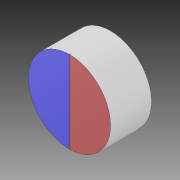
# Autodesk Inventor part: DiametricMagnet 1-4 x 1-8
Saved by Autodesk Inventor 2020 (Build 240168000, 168)
## iProperties
Created: 2021-06-12
Part Number: DiametricMagnet 1-4 x 1-8
Material: Generic
Document SubType Name: Modeling
Designer: DDeGo
Density: 1 g/cm^3
Appearance: Default
Author: DDeGo
Autodesk Inventor part; units mm, degrees
ref_plane "YZ Plane" through (0, 0, 0) normal (1, 0, 0) x (0, 1, 0)
ref_plane "XZ Plane" through (0, 0, 0) normal (0, 1, 0) x (-1, 0, 0)
ref_plane "XY Plane" through (0, 0, 0) normal (0, 0, 1) x (1, 0, 0)
sketch "Sketch1" plane through (0, 0, 0) normal (0, 0, 1) x (1, 0, 0)
  circle A0 centre (0, 0) radius 3.175
  dimension "d0" = 6.35
  constraints: 1 centre point, 1 coincident
  measures "d0" diameter of A0
extrude "Extrusion1" add sketch "Sketch1" along normal blind 3.175
sketch "Sketch2" plane through (0, 0, 3.175) normal (0, 0, 1) x (1, 0, 0)
  line L0 (-0.005, 4.4092) -> (0.005, 4.4092)
  line L1 (0.005, 4.4092) -> (0.005, -4.4092)
  line L2 (0.005, -4.4092) -> (-0.005, -4.4092)
  line L3 (-0.005, -4.4092) -> (-0.005, 4.4092)
  line L4 (-0.005, 4.4092) -> (0.005, -4.4092) construction
  line L5 (0.005, 4.4092) -> (-0.005, -4.4092) construction
  point P0 (0, 0)
  dimension "d3" = 8.8185
  dimension "d4" = 0.01
  constraints: 12 end point, 2 midpoint, 2 parallel, 1 horizontal, 1 perpendicular
  measures "d3" distance of L2.end L0.start
  measures "d4" distance between parallel lines of L1 L3
extrude "Extrusion2" cut sketch "Sketch2" against normal blind 0.1
body "Solid1"
